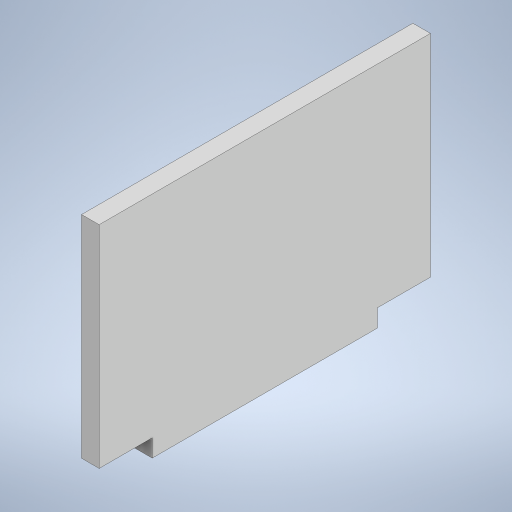
# Autodesk Inventor part: servo long side
Saved by Autodesk Inventor 2023 (Build 270158000, 158)
## iProperties
Created: 2023-10-15
Part Number: servo long side
Material: Generic
Document SubType Name: Modeling
Designer: Nate
Density: 1 g/cm^3
Appearance: Default
Author: Nate
Autodesk Inventor part; units mm, degrees
ref_plane "YZ Plane" through (0, 0, 0) normal (1, 0, 0) x (0, 1, 0)
ref_plane "XZ Plane" through (0, 0, 0) normal (0, 1, 0) x (-1, 0, 0)
ref_plane "XY Plane" through (0, 0, 0) normal (0, 0, 1) x (1, 0, 0)
sketch "Sketch1" plane through (0, 0, 0) normal (0, 0, 1) x (1, 0, 0)
  line L0 (0, 0) -> (-3.175, 0)
  line L1 (-3.175, 0) -> (-3.175, 40.64)
  line L2 (-3.175, 40.64) -> (0, 40.64)
  line L3 (0, 40.64) -> (0, 0)
  line L4 (-41.275, -9.5758) -> (-3.175, -9.5758)
  line L5 (-3.175, -9.5758) -> (-3.175, 50.2158)
  line L6 (-3.175, 50.2158) -> (-41.275, 50.2158)
  line L7 (-41.275, 50.2158) -> (-41.275, -9.5758)
  point P0 (-22.225, 50.2158)
  point P1 (-22.225, -9.5758)
  point P2 (-3.175, 0)
  point P3 (-3.175, 40.64)
  dimension "d0" = 3.175
  dimension "d1" = 40.64
  dimension "d2" = 59.7916
  dimension "d3" = 9.5758
  dimension "d5" = 38.1
  dimension "d6" = 0
  constraints: 16 end point, 4 parallel, 2 horizontal, 2 midpoint, 2 perpendicular
  measures "d0" distance of L1.end L2.end
  measures "d1" distance of L0.end L1.end
  measures "d2" distance of point (-22.225, 50.216) point (-22.225, -9.576)
  measures "d3" distance between parallel lines of L0 L4
  measures "d5" distance between parallel lines of L7 L1
  measures "d6" distance between parallel lines of L1 L5
extrude "Extrusion1" add sketch "Sketch1" along normal blind 3.175
move or copy body "Move Body1" bodies to move or copy 1 copy no rotation origin (0, 0, 0) rotation axis (0, 0, 1) rotation angle -90 translate (-40.64, 40.64, 0)
move or copy body "Move Body2" bodies to move or copy 1 copy no rotation origin (0, 0, 0) rotation axis (0, -1, 0) rotation angle -90 translate (9.5758, 0, 9.5758)
move or copy body "Move Body3" bodies to move or copy 1 copy no translate (25.4, 0, 0)
body "Solid1"
